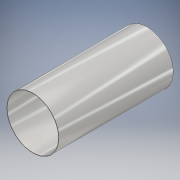
# Autodesk Inventor part: DPLX_P008_Wire_Mesh_Sleeve_Trans
Saved by Autodesk Inventor 2018 (Build 220112000, 112)
## iProperties
Created: 2018-06-07
Part Number: DPLX_P008_Wire_Mesh_Sleeve_Trans
Material: Aluminum 6061
Document SubType Name: Modeling
Designer: DPLXuser
Density: 2.7 g/cm^3
Appearance: Aluminum - Polished
Author: DPLXuser
Autodesk Inventor part; units mm, degrees
ref_plane "YZ Plane" through (0, 0, 0) normal (1, 0, 0) x (0, 1, 0)
ref_plane "XZ Plane" through (0, 0, 0) normal (0, 1, 0) x (-1, 0, 0)
ref_plane "XY Plane" through (0, 0, 0) normal (0, 0, 1) x (1, 0, 0)
sketch "Sketch1" plane through (0, 0, 0) normal (0, 1, 0) x (-1, 0, 0)
  circle A0 centre (0, 0) radius 15.6718
  circle A1 centre (0, 0) radius 15.9383
  dimension "d0" = 31.3436
  dimension "d1" = 31.8766
  constraints: 2 centre point, 2 coincident
  measures "d0" diameter of A0
  measures "d1" diameter of A1
extrude "Extrusion1" add sketch "Sketch1" along normal blind 70
sketch "Sketch2" plane through (0, 0, 0) normal (0, -1, 0) x (1, 0, 0)
  point P0 (0, 0)
body "Solid1"
